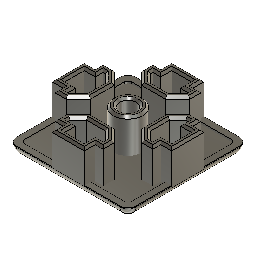
EXTRUSIONcap (Autodesk Fusion 360 design; units mm, degrees)
Autodesk Fusion 360 part; units mm, degrees
sketch "Sketch1" plane through (0, 0, 0) normal (0, 0, 1) x (1, 0, 0)
  line L0 (15, 15) -> (-15, 15)
  line L1 (-15, 15) -> (-15, -15)
  line L2 (-15, -15) -> (15, -15)
  line L3 (15, -15) -> (15, 15)
  line L4 (15, 15) -> (-15, -15) construction
  line L5 (-15, 15) -> (15, -15) construction
  line L6 (0, -15) -> (0, 15) construction
  line L7 (15, 0) -> (-15, 0) construction
  line L8 (-4, -15) -> (4, -15)
  line L9 (4, -15) -> (4, -6.5)
  line L10 (4, -6.5) -> (-4, -6.5)
  line L11 (-4, -6.5) -> (-4, -15)
  line L12 (-4, -15) -> (4, -6.5) construction
  line L13 (4, -15) -> (-4, -6.5) construction
  circle A0 centre (0, 0) radius 3.65
  line L14 (-3, -6.5) -> (3, -6.5)
  line L15 (6, -9.5) -> (6, -12.25)
  line L16 (6, -12.25) -> (-6, -12.25) construction
  line L17 (-6, -12.25) -> (-6, -9.5)
  line L18 (-6, -6.5) -> (6, -12.25) construction
  line L19 (6, -6.5) -> (-6, -12.25) construction
  line L20 (-6, -12.25) -> (-4, -12.25)
  line L21 (-4, -15) -> (-4, -12.25)
  line L22 (6, -12.25) -> (4, -12.25)
  line L23 (4, -12.25) -> (4, -15)
  line L24 (-6, -9.5) -> (-3, -6.5)
  line L25 (3, -6.5) -> (6, -9.5)
  point P0 (0, -10.75)
  point P1 (0, -9.375)
  dimension "d13" = 30
  dimension "d14" = 30
  dimension "d19" = 8
  dimension "d20" = 8.5
  dimension "d23" = 7.3
  dimension "d45" = 12
  dimension "d46" = 5.75
  dimension "d52" = 3
  dimension "d53" = 3
  dimension "d54" = 3
  dimension "d55" = 3
  constraint horizontal L0
  constraint perpendicular L0 L1
  constraint parallel L0 L2
  constraint parallel L1 L3
  constraint coincident L4 A0.centre
  constraint coincident L5 A0.centre
  constraint coincident A0.centre origin
  constraint midpoint L2 L6.start
  constraint midpoint L0 L6.end
  constraint midpoint L3 L7.start
  constraint midpoint L1 L7.end
  constraint horizontal L8
  constraint perpendicular L8 L9
  constraint parallel L8 L10
  constraint parallel L9 L11
  constraint coincident L12 P0
  constraint coincident L13 P0
  constraint coincident L6 P0
  constraint collinear L2 L8
  constraint horizontal L14
  constraint perpendicular L14 L15
  constraint parallel L14 L16
  constraint parallel L15 L17
  constraint coincident L18 P1
  constraint coincident L19 P1
  constraint coincident L6 P1
  constraint collinear L10 L14
  constraint coincident L16 L20.end
  constraint coincident L11 L20.end
  constraint coincident L16 L22.end
  constraint coincident L9 L22.end
  constraint coincident L18.start L17
  constraint coincident L18.start L14
  constraint coincident L19.start L14
  constraint coincident L19.start L15
  measures "d13" distance of L1.end L2.end
  measures "d14" distance of L0.end L1.end
  measures "d19" distance of L9.end L10.end
  measures "d20" distance of L8.end L9.end
  measures "d23" diameter of A0
  measures "d45" distance of L15.end L16.end
  measures "d46" distance of L19.start L15.end
  measures "d52" distance of L18.start L17.end
  measures "d53" distance of L18.start L14.start
  measures "d54" distance of L19.start L14.end
  measures "d55" distance of L19.start L15.start
extrude "Extrude1" add sketch "Sketch1" along normal blind 2 thin wall 1.5 inside contours L0 L1 L2 L3 L9 L10 L11 L14 L15 L17 L20 L21 L22 L23 L24 L25 | L2 L8 L9 L10 L11 L14 L21 L23 L24 L25 | L9 L15 L22 L25 | L11 L17 L20 L24 | L9 L10 L25 | L10 L11 L24 | A0 in component "foot"
extrude "Extrude3" add sketch "Sketch1" along normal blind 1.5 contours L0 L1 L2 L3 L9 L10 L11 L14 L15 L17 L20 L21 L22 L23 L24 L25 | L2 L8 L9 L10 L11 L14 L21 L23 L24 L25 | L9 L15 L22 L25 | L11 L17 L20 L24 | L9 L10 L25 | L10 L11 L24 | A0 in component "foot"
extrude "Extrude4" add sketch "Sketch1" along normal blind 8.5 from surface at 1.5 thin wall 1.5 inside contours A0 in component "foot"
extrude "Extrude2" add sketch "Sketch1" along normal blind 8.5 from surface at 1.5 thin wall 1.5 inside contours L2 L8 L9 L10 L11 L14 L21 L23 L24 L25 | L9 L15 L22 L25 | L11 L17 L20 L24 in component "foot"
chamfer "Chamfer3" distance 0.5 angle 45 1 faces at (0.8333, -14.5, 10) in component "foot"
fillet "Fillet1" radius 2 4 edges at (-15, -15, 1) (15, -15, 1) (15, 15, 1) (-15, 15, 1) in component "foot"
fillet "Fillet1" radius 1 4 edges at (-13.5, -13.5, 1.75) (-13.5, 13.5, 1.75) (13.5, -13.5, 1.75) (13.5, 13.5, 1.75) in component "foot"
chamfer "Chamfer1" distance 1 angle 45 8 edges at (0, 15, 0) (-14.4142, 14.4142, 0) (-15, 0, 0) (-14.4142, -14.4142, 0) (0, -15, 0) (14.4142, -14.4142, 0) (15, 0, 0) (14.4142, 14.4142, 0) in component "foot"
chamfer "Chamfer1" distance 0.5 angle 45 1 faces at (3.1284, -0.2881, 10) in component "foot"
fillet "Fillet3" radius 2 8 edges at (-15, 0, 1) (-14.4142, 14.4142, 1) (0, 15, 1) (14.4142, 14.4142, 1) (15, 0, 1) (14.4142, -14.4142, 1) (0, -15, 1) (-14.4142, -14.4142, 1) in component "foot"
pattern_circular "C-Pattern1" count 4 over 360 about axis through (0, 0, 1.75) along (0, 0, 1) of "Extrude2", "Chamfer3" in component "foot"
component "foot" placed x (1, 0, 0) y (0, 1, 0) z (0, 0, 1) at (0, 0, 0)
equation "d15 = heightCap"
equation "d24 = heightTotal - 1.5 mm"
equation "heightCap = 2 mm"
equation "d53 = d52"
equation "d55 = d54"
equation "d58 = heightTotal - 1.5 mm"
equation "heightTotal = 10 mm"
